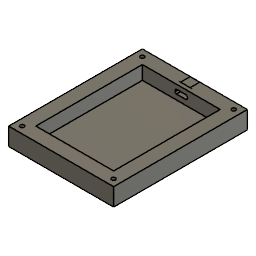
Bottom (Autodesk Fusion 360 design; units mm, degrees)
Autodesk Fusion 360 part; units mm, degrees
sketch "Sketch1" plane through (0, 0, 0) normal (0, 1, 0) x (1, 0, 0)
  line L0 (0, 0) -> (56.985, 0)
  line L1 (56.985, 0) -> (56.985, 78.065)
  line L2 (56.985, 78.065) -> (0, 78.065)
  line L3 (0, 78.065) -> (0, 0)
  line L4 (66.985, -10) -> (66.985, 88.065)
  line L5 (66.985, 88.065) -> (-10, 88.065)
  line L6 (-10, 88.065) -> (-10, -10)
  line L7 (-10, -10) -> (66.985, -10)
  circle A0 centre (-5, 83.065) radius 1.45
  circle A1 centre (-5, -5) radius 1.45
  circle A2 centre (61.985, -5) radius 1.45
  circle A3 centre (61.985, 83.065) radius 1.45
  dimension "d4" = 56.985
  dimension "d5" = 78.065
  dimension "d6" = 10
  dimension "d9" = 2.9
  dimension "d12" = 2.9
  dimension "d15" = 2.9
  dimension "d18" = 2.9
  constraint horizontal L0
  constraint vertical L1
  constraint horizontal L2
  constraint vertical L3
  constraint coincident L0.start L3.end
  measures "d4" distance of L0.start L0.end
  measures "d5" distance of L0.start L2.end
  measures "d9" diameter of A0
  measures "d12" diameter of A1
  measures "d15" diameter of A2
  measures "d18" diameter of A3
extrude "Extrude1" add sketch "Sketch1" along normal blind 3 contours L0 L1 L2 L3 | L4 L5 L6 L7 picked at (18.995, 52.043333) picked at (60.825164, 26.021667) makes body 1
extrude "Extrude2" cut sketch "Sketch1" along normal blind 13 bodies 1
extrude "Extrude3" add sketch "Sketch1" along normal blind 13 bodies 1
move_body "Align1" bodies 1 to x (1, 0, 0) y (0, 1, 0) z (0, 0, 1) at (0, 0, 0)
move_body "Align2" bodies 1 to x (1, 0, 0) y (0, 1, 0) z (0, 0, 1) at (0, 0, 0)
move_body "Align3" bodies 1 to x (1, 0, 0) y (0, 1, 0) z (0, 0, 1) at (-28.4925, -5.248423, 39.0325)
sketch "plate-2026-03-13T21_26_14.409Z" plane through (0, 7.751577, 0) normal (0, 1, 0) x (1, 0, 0)
  line L0 (-25.209257, 35.572548) -> (-12.209257, 35.572548)
  line L1 (-25.209257, 21.572548) -> (-12.209257, 21.572548)
  line L2 (-25.709257, 35.072548) -> (-25.709257, 22.072548)
  line L3 (-11.709257, 35.072548) -> (-11.709257, 22.072548)
  arc A0 (-25.209257, 35.572548) -> (-25.709257, 35.072548) centre (-25.209257, 35.072548) ccw
  arc A1 (-11.709257, 35.072548) -> (-12.209257, 35.572548) centre (-12.209257, 35.072548) ccw
  arc A2 (-25.709257, 22.072548) -> (-25.209257, 21.572548) centre (-25.209257, 22.072548) ccw
  arc A3 (-12.209257, 21.572548) -> (-11.709257, 22.072548) centre (-12.209257, 22.072548) ccw
  line L4 (-6.159257, 35.572548) -> (6.840743, 35.572548)
  line L5 (-6.159257, 21.572548) -> (6.840743, 21.572548)
  line L6 (-6.659257, 35.072548) -> (-6.659257, 22.072548)
  line L7 (7.340743, 35.072548) -> (7.340743, 22.072548)
  arc A4 (-6.159257, 35.572548) -> (-6.659257, 35.072548) centre (-6.159257, 35.072548) ccw
  arc A5 (7.340743, 35.072548) -> (6.840743, 35.572548) centre (6.840743, 35.072548) ccw
  arc A6 (-6.659257, 22.072548) -> (-6.159257, 21.572548) centre (-6.159257, 22.072548) ccw
  arc A7 (6.840743, 21.572548) -> (7.340743, 22.072548) centre (6.840743, 22.072548) ccw
  line L8 (12.890743, 35.572548) -> (25.890743, 35.572548)
  line L9 (12.890743, 21.572548) -> (25.890743, 21.572548)
  line L10 (12.390743, 35.072548) -> (12.390743, 22.072548)
  line L11 (26.390743, 35.072548) -> (26.390743, 22.072548)
  arc A8 (12.890743, 35.572548) -> (12.390743, 35.072548) centre (12.890743, 35.072548) ccw
  arc A9 (26.390743, 35.072548) -> (25.890743, 35.572548) centre (25.890743, 35.072548) ccw
  arc A10 (12.390743, 22.072548) -> (12.890743, 21.572548) centre (12.890743, 22.072548) ccw
  arc A11 (25.890743, 21.572548) -> (26.390743, 22.072548) centre (25.890743, 22.072548) ccw
  line L12 (-25.209257, 16.522548) -> (-12.209257, 16.522548)
  line L13 (-25.209257, 2.522548) -> (-12.209257, 2.522548)
  line L14 (-25.709257, 16.022548) -> (-25.709257, 3.022548)
  line L15 (-11.709257, 16.022548) -> (-11.709257, 3.022548)
  arc A12 (-25.209257, 16.522548) -> (-25.709257, 16.022548) centre (-25.209257, 16.022548) ccw
  arc A13 (-11.709257, 16.022548) -> (-12.209257, 16.522548) centre (-12.209257, 16.022548) ccw
  arc A14 (-25.709257, 3.022548) -> (-25.209257, 2.522548) centre (-25.209257, 3.022548) ccw
  arc A15 (-12.209257, 2.522548) -> (-11.709257, 3.022548) centre (-12.209257, 3.022548) ccw
  line L16 (-6.159257, 16.522548) -> (6.840743, 16.522548)
  line L17 (-6.159257, 2.522548) -> (6.840743, 2.522548)
  line L18 (-6.659257, 16.022548) -> (-6.659257, 3.022548)
  line L19 (7.340743, 16.022548) -> (7.340743, 3.022548)
  arc A16 (-6.159257, 16.522548) -> (-6.659257, 16.022548) centre (-6.159257, 16.022548) ccw
  arc A17 (7.340743, 16.022548) -> (6.840743, 16.522548) centre (6.840743, 16.022548) ccw
  arc A18 (-6.659257, 3.022548) -> (-6.159257, 2.522548) centre (-6.159257, 3.022548) ccw
  arc A19 (6.840743, 2.522548) -> (7.340743, 3.022548) centre (6.840743, 3.022548) ccw
  line L20 (12.890743, 16.522548) -> (25.890743, 16.522548)
  line L21 (12.890743, 2.522548) -> (25.890743, 2.522548)
  line L22 (12.390743, 16.022548) -> (12.390743, 3.022548)
  line L23 (26.390743, 16.022548) -> (26.390743, 3.022548)
  arc A20 (12.890743, 16.522548) -> (12.390743, 16.022548) centre (12.890743, 16.022548) ccw
  arc A21 (26.390743, 16.022548) -> (25.890743, 16.522548) centre (25.890743, 16.022548) ccw
  arc A22 (12.390743, 3.022548) -> (12.890743, 2.522548) centre (12.890743, 3.022548) ccw
  arc A23 (25.890743, 2.522548) -> (26.390743, 3.022548) centre (25.890743, 3.022548) ccw
  line L24 (-25.209257, -2.527452) -> (-12.209257, -2.527452)
  line L25 (-25.209257, -16.527452) -> (-12.209257, -16.527452)
  line L26 (-25.709257, -3.027452) -> (-25.709257, -16.027452)
  line L27 (-11.709257, -3.027452) -> (-11.709257, -16.027452)
  arc A24 (-25.209257, -2.527452) -> (-25.709257, -3.027452) centre (-25.209257, -3.027452) ccw
  arc A25 (-11.709257, -3.027452) -> (-12.209257, -2.527452) centre (-12.209257, -3.027452) ccw
  arc A26 (-25.709257, -16.027452) -> (-25.209257, -16.527452) centre (-25.209257, -16.027452) ccw
  arc A27 (-12.209257, -16.527452) -> (-11.709257, -16.027452) centre (-12.209257, -16.027452) ccw
  line L28 (-6.159257, -2.527452) -> (6.840743, -2.527452)
  line L29 (-6.159257, -16.527452) -> (6.840743, -16.527452)
  line L30 (-6.659257, -3.027452) -> (-6.659257, -16.027452)
  line L31 (7.340743, -3.027452) -> (7.340743, -16.027452)
  arc A28 (-6.159257, -2.527452) -> (-6.659257, -3.027452) centre (-6.159257, -3.027452) ccw
  arc A29 (7.340743, -3.027452) -> (6.840743, -2.527452) centre (6.840743, -3.027452) ccw
  arc A30 (-6.659257, -16.027452) -> (-6.159257, -16.527452) centre (-6.159257, -16.027452) ccw
  arc A31 (6.840743, -16.527452) -> (7.340743, -16.027452) centre (6.840743, -16.027452) ccw
  line L32 (12.890743, -2.527452) -> (25.890743, -2.527452)
  line L33 (12.890743, -16.527452) -> (25.890743, -16.527452)
  line L34 (12.390743, -3.027452) -> (12.390743, -16.027452)
  line L35 (26.390743, -3.027452) -> (26.390743, -16.027452)
  arc A32 (12.890743, -2.527452) -> (12.390743, -3.027452) centre (12.890743, -3.027452) ccw
  arc A33 (26.390743, -3.027452) -> (25.890743, -2.527452) centre (25.890743, -3.027452) ccw
  arc A34 (12.390743, -16.027452) -> (12.890743, -16.527452) centre (12.890743, -16.027452) ccw
  arc A35 (25.890743, -16.527452) -> (26.390743, -16.027452) centre (25.890743, -16.027452) ccw
  line L36 (12.890743, -2.527452) -> (25.890743, -2.527452)
  line L37 (12.890743, -16.527452) -> (25.890743, -16.527452)
  line L38 (12.390743, -3.027452) -> (12.390743, -16.027452)
  line L39 (26.390743, -3.027452) -> (26.390743, -16.027452)
  arc A36 (12.890743, -2.527452) -> (12.390743, -3.027452) centre (12.890743, -3.027452) ccw
  arc A37 (26.390743, -3.027452) -> (25.890743, -2.527452) centre (25.890743, -3.027452) ccw
  arc A38 (12.390743, -16.027452) -> (12.890743, -16.527452) centre (12.890743, -16.027452) ccw
  arc A39 (25.890743, -16.527452) -> (26.390743, -16.027452) centre (25.890743, -16.027452) ccw
  line L40 (-25.209257, -21.577452) -> (-12.209257, -21.577452)
  line L41 (-25.209257, -35.577452) -> (-12.209257, -35.577452)
  line L42 (-25.709257, -22.077452) -> (-25.709257, -35.077452)
  line L43 (-11.709257, -22.077452) -> (-11.709257, -35.077452)
  arc A40 (-25.209257, -21.577452) -> (-25.709257, -22.077452) centre (-25.209257, -22.077452) ccw
  arc A41 (-11.709257, -22.077452) -> (-12.209257, -21.577452) centre (-12.209257, -22.077452) ccw
  arc A42 (-25.709257, -35.077452) -> (-25.209257, -35.577452) centre (-25.209257, -35.077452) ccw
  arc A43 (-12.209257, -35.577452) -> (-11.709257, -35.077452) centre (-12.209257, -35.077452) ccw
  line L44 (-6.159257, -21.577452) -> (6.840743, -21.577452)
  line L45 (-6.159257, -35.577452) -> (6.840743, -35.577452)
  line L46 (-6.659257, -22.077452) -> (-6.659257, -35.077452)
  line L47 (7.340743, -22.077452) -> (7.340743, -35.077452)
  arc A44 (-6.159257, -21.577452) -> (-6.659257, -22.077452) centre (-6.159257, -22.077452) ccw
  arc A45 (7.340743, -22.077452) -> (6.840743, -21.577452) centre (6.840743, -22.077452) ccw
  arc A46 (-6.659257, -35.077452) -> (-6.159257, -35.577452) centre (-6.159257, -35.077452) ccw
  arc A47 (6.840743, -35.577452) -> (7.340743, -35.077452) centre (6.840743, -35.077452) ccw
  line L48 (12.890743, -21.577452) -> (25.890743, -21.577452)
  line L49 (12.890743, -35.577452) -> (25.890743, -35.577452)
  line L50 (12.390743, -22.077452) -> (12.390743, -35.077452)
  line L51 (26.390743, -22.077452) -> (26.390743, -35.077452)
  arc A48 (12.890743, -21.577452) -> (12.390743, -22.077452) centre (12.890743, -22.077452) ccw
  arc A49 (26.390743, -22.077452) -> (25.890743, -21.577452) centre (25.890743, -22.077452) ccw
  arc A50 (12.390743, -35.077452) -> (12.890743, -35.577452) centre (12.890743, -35.077452) ccw
  arc A51 (25.890743, -35.577452) -> (26.390743, -35.077452) centre (25.890743, -35.077452) ccw
  line L52 (-28.234257, -39.156471) -> (28.915743, -39.156471)
  line L53 (-28.234257, 39.046164) -> (28.915743, 39.046164)
  line L54 (-28.234257, -39.156471) -> (-28.234257, 39.046164)
  line L55 (28.915743, -39.156471) -> (28.915743, 39.046164)
move_body "Move1" bodies 1 to x (1, 0, 0) y (0, 1, 0) z (0, 0, 1) at (0.258, 0, 0)
extrude "Extrude4" add sketch "plate-2026-03-13T21_26_14.409Z" 1 faces at (32.590664, 7.751577, 13.010833) along normal blind 3 separate body on bodies 1 makes body 2
sketch "Sketch3" plane through (0, 0, -49.0325) normal (0, 0, -1) x (-1, 0, 0)
  line L0 (-38.7505, -5.248423) -> (38.2345, -5.248423)
  line L1 (38.2345, -5.248423) -> (38.2345, 7.751577)
  line L2 (38.2345, 7.751577) -> (-38.7505, 7.751577)
  line L3 (-38.7505, 7.751577) -> (-38.7505, -5.248423)
  line L4 (-3.758, 1.551577) -> (3.242, 1.551577)
  line L5 (4.242, 2.551577) -> (4.242, 3.551577)
  line L6 (3.242, 4.551577) -> (-3.758, 4.551577)
  line L7 (-4.758, 3.551577) -> (-4.758, 2.551577)
  arc A0 (4.242, 3.551577) -> (3.242, 4.551577) centre (3.242, 3.551577) ccw
  arc A1 (3.242, 1.551577) -> (4.242, 2.551577) centre (3.242, 2.551577) ccw
  arc A2 (-3.758, 4.551577) -> (-4.758, 3.551577) centre (-3.758, 3.551577) ccw
  arc A3 (-4.758, 2.551577) -> (-3.758, 1.551577) centre (-3.758, 2.551577) ccw
  dimension "d34" = 1
  dimension "d35" = 1
  dimension "d36" = 1
  dimension "d37" = 1
  constraint horizontal L4
  constraint vertical L5
  constraint horizontal L6
  constraint vertical L7
  constraint tangent L6 A0
  constraint tangent L5 A0
  constraint tangent L4 A1
  constraint tangent L5 A1
  constraint tangent L7 A2
  constraint tangent L6 A2
  constraint tangent L7 A3
  constraint tangent L4 A3
  measures "d34" radius of A0
  measures "d35" radius of A1
  measures "d36" radius of A2
  measures "d37" radius of A3
extrude "Extrude5" cut sketch "Sketch3" against normal blind 17 contours L4 L5 L6 L7 A0 A1 A2 A3 picked at (0.908667, 2.551577) bodies 1
sketch "Sketch4" plane through (0, 0, -49.0325) normal (0, 0, -1) x (-1, 0, 0)
  line L0 (3.242, 1.551577) -> (-3.758, 1.551577)
  arc A0 (-4.758, 2.551577) -> (-3.758, 1.551577) centre (-3.758, 2.551577) ccw
  line L1 (-4.758, 2.551577) -> (-4.758, 3.551577)
  arc A1 (-3.758, 4.551577) -> (-4.758, 3.551577) centre (-3.758, 3.551577) ccw
  line L2 (-3.758, 4.551577) -> (3.242, 4.551577)
  arc A2 (4.242, 3.551577) -> (3.242, 4.551577) centre (3.242, 3.551577) ccw
  line L3 (4.242, 3.551577) -> (4.242, 2.551577)
  arc A3 (3.242, 1.551577) -> (4.242, 2.551577) centre (3.242, 2.551577) ccw
  line L4 (-38.7505, -5.248423) -> (38.2345, -5.248423)
  line L5 (38.2345, -5.248423) -> (38.2345, 7.751577)
  line L6 (38.2345, 7.751577) -> (-38.7505, 7.751577)
  line L7 (-38.7505, 7.751577) -> (-38.7505, -5.248423)
  arc A4 (7.242, 3.551577) -> (3.242, 7.551577) centre (3.242, 3.551577) ccw
  line L8 (-3.758, 7.551577) -> (3.242, 7.551577)
  arc A5 (-3.758, 7.551577) -> (-7.758, 3.551577) centre (-3.758, 3.551577) ccw
  line L9 (-7.758, 2.551577) -> (-7.758, 3.551577)
  arc A6 (-7.758, 2.551577) -> (-3.758, -1.448423) centre (-3.758, 2.551577) ccw
  line L10 (3.242, -1.448423) -> (-3.758, -1.448423)
  arc A7 (3.242, -1.448423) -> (7.242, 2.551577) centre (3.242, 2.551577) ccw
  line L11 (7.242, 3.551577) -> (7.242, 2.551577)
  dimension "d40" = -3
extrude "Extrude6" cut sketch "Sketch4" against normal blind 7 contours A4 L8 A5 L9 A6 L10 A7 L11 picked at (-1.424667, -0.448423) bodies 1
sketch "Sketch5" plane through (38.7505, 0, 0) normal (1, 0, 0) x (0, 0, -1)
  line L0 (-49.0325, 7.751577) -> (49.0325, 7.751577)
  line L1 (49.0325, 7.751577) -> (49.0325, 10.751577)
  line L2 (49.0325, 10.751577) -> (-49.0325, 10.751577)
  line L3 (-49.0325, 10.751577) -> (-49.0325, 7.751577)
  line L4 (-49.0325, 9.251577) -> (49.0325, 9.251577)
extrude "Extrude7" cut sketch "Sketch5" against normal blind 88 contours L1 L2 L3 L4 picked at (-16.344167, 10.251577) bodies 2
sketch "Sketch6" plane through (0, 9.251577, 0) normal (0, 1, 0) x (-1, 0, 0)
  line L0 (38.2345, -49.0325) -> (38.2345, 49.0325)
  line L1 (38.2345, 49.0325) -> (-38.7505, 49.0325)
  line L2 (-38.7505, 49.0325) -> (-38.7505, -49.0325)
  line L3 (-38.7505, -49.0325) -> (38.2345, -49.0325)
  line L4 (-12.390743, 16.027452) -> (-12.390743, 3.027452)
  arc A0 (-12.890743, 2.527452) -> (-12.390743, 3.027452) centre (-12.890743, 3.027452) ccw
  line L5 (-12.890743, 2.527452) -> (-25.890743, 2.527452)
  arc A1 (-26.390743, 3.027452) -> (-25.890743, 2.527452) centre (-25.890743, 3.027452) ccw
  line L6 (-26.390743, 3.027452) -> (-26.390743, 16.027452)
  arc A2 (-25.890743, 16.527452) -> (-26.390743, 16.027452) centre (-25.890743, 16.027452) ccw
  line L7 (-25.890743, 16.527452) -> (-12.890743, 16.527452)
  arc A3 (-12.390743, 16.027452) -> (-12.890743, 16.527452) centre (-12.890743, 16.027452) ccw
  line L8 (25.709257, -3.022548) -> (25.709257, -16.022548)
  arc A4 (25.209257, -16.522548) -> (25.709257, -16.022548) centre (25.209257, -16.022548) ccw
  line L9 (25.209257, -16.522548) -> (12.209257, -16.522548)
  arc A5 (11.709257, -16.022548) -> (12.209257, -16.522548) centre (12.209257, -16.022548) ccw
  line L10 (11.709257, -16.022548) -> (11.709257, -3.022548)
  arc A6 (12.209257, -2.522548) -> (11.709257, -3.022548) centre (12.209257, -3.022548) ccw
  line L11 (12.209257, -2.522548) -> (25.209257, -2.522548)
  arc A7 (25.709257, -3.022548) -> (25.209257, -2.522548) centre (25.209257, -3.022548) ccw
  line L12 (-12.390743, 35.077452) -> (-12.390743, 22.077452)
  arc A8 (-12.890743, 21.577452) -> (-12.390743, 22.077452) centre (-12.890743, 22.077452) ccw
  line L13 (-12.890743, 21.577452) -> (-25.890743, 21.577452)
  arc A9 (-26.390743, 22.077452) -> (-25.890743, 21.577452) centre (-25.890743, 22.077452) ccw
  line L14 (-26.390743, 22.077452) -> (-26.390743, 35.077452)
  arc A10 (-25.890743, 35.577452) -> (-26.390743, 35.077452) centre (-25.890743, 35.077452) ccw
  line L15 (-25.890743, 35.577452) -> (-12.890743, 35.577452)
  arc A11 (-12.390743, 35.077452) -> (-12.890743, 35.577452) centre (-12.890743, 35.077452) ccw
  line L16 (6.659257, 16.027452) -> (6.659257, 3.027452)
  arc A12 (6.159257, 2.527452) -> (6.659257, 3.027452) centre (6.159257, 3.027452) ccw
  line L17 (6.159257, 2.527452) -> (-6.840743, 2.527452)
  arc A13 (-7.340743, 3.027452) -> (-6.840743, 2.527452) centre (-6.840743, 3.027452) ccw
  line L18 (-7.340743, 3.027452) -> (-7.340743, 16.027452)
  arc A14 (-6.840743, 16.527452) -> (-7.340743, 16.027452) centre (-6.840743, 16.027452) ccw
  line L19 (-6.840743, 16.527452) -> (6.159257, 16.527452)
  arc A15 (6.659257, 16.027452) -> (6.159257, 16.527452) centre (6.159257, 16.027452) ccw
  line L20 (25.709257, 16.027452) -> (25.709257, 3.027452)
  arc A16 (25.209257, 2.527452) -> (25.709257, 3.027452) centre (25.209257, 3.027452) ccw
  line L21 (25.209257, 2.527452) -> (12.209257, 2.527452)
  arc A17 (11.709257, 3.027452) -> (12.209257, 2.527452) centre (12.209257, 3.027452) ccw
  line L22 (11.709257, 3.027452) -> (11.709257, 16.027452)
  arc A18 (12.209257, 16.527452) -> (11.709257, 16.027452) centre (12.209257, 16.027452) ccw
  line L23 (12.209257, 16.527452) -> (25.209257, 16.527452)
  arc A19 (25.709257, 16.027452) -> (25.209257, 16.527452) centre (25.209257, 16.027452) ccw
  line L24 (6.659257, 35.077452) -> (6.659257, 22.077452)
  arc A20 (6.159257, 21.577452) -> (6.659257, 22.077452) centre (6.159257, 22.077452) ccw
  line L25 (6.159257, 21.577452) -> (-6.840743, 21.577452)
  arc A21 (-7.340743, 22.077452) -> (-6.840743, 21.577452) centre (-6.840743, 22.077452) ccw
  line L26 (-7.340743, 22.077452) -> (-7.340743, 35.077452)
  arc A22 (-6.840743, 35.577452) -> (-7.340743, 35.077452) centre (-6.840743, 35.077452) ccw
  line L27 (-6.840743, 35.577452) -> (6.159257, 35.577452)
  arc A23 (6.659257, 35.077452) -> (6.159257, 35.577452) centre (6.159257, 35.077452) ccw
  line L28 (-12.390743, -3.022548) -> (-12.390743, -16.022548)
  arc A24 (-12.890743, -16.522548) -> (-12.390743, -16.022548) centre (-12.890743, -16.022548) ccw
  line L29 (-12.890743, -16.522548) -> (-25.890743, -16.522548)
  arc A25 (-26.390743, -16.022548) -> (-25.890743, -16.522548) centre (-25.890743, -16.022548) ccw
  line L30 (-26.390743, -16.022548) -> (-26.390743, -3.022548)
  arc A26 (-25.890743, -2.522548) -> (-26.390743, -3.022548) centre (-25.890743, -3.022548) ccw
  line L31 (-25.890743, -2.522548) -> (-12.890743, -2.522548)
  arc A27 (-12.390743, -3.022548) -> (-12.890743, -2.522548) centre (-12.890743, -3.022548) ccw
  line L32 (-12.390743, -22.072548) -> (-12.390743, -35.072548)
  arc A28 (-12.890743, -35.572548) -> (-12.390743, -35.072548) centre (-12.890743, -35.072548) ccw
  line L33 (-12.890743, -35.572548) -> (-25.890743, -35.572548)
  arc A29 (-26.390743, -35.072548) -> (-25.890743, -35.572548) centre (-25.890743, -35.072548) ccw
  line L34 (-26.390743, -35.072548) -> (-26.390743, -22.072548)
  arc A30 (-25.890743, -21.572548) -> (-26.390743, -22.072548) centre (-25.890743, -22.072548) ccw
  line L35 (-25.890743, -21.572548) -> (-12.890743, -21.572548)
  arc A31 (-12.390743, -22.072548) -> (-12.890743, -21.572548) centre (-12.890743, -22.072548) ccw
  line L36 (6.659257, -3.022548) -> (6.659257, -16.022548)
  arc A32 (6.159257, -16.522548) -> (6.659257, -16.022548) centre (6.159257, -16.022548) ccw
  line L37 (6.159257, -16.522548) -> (-6.840743, -16.522548)
  arc A33 (-7.340743, -16.022548) -> (-6.840743, -16.522548) centre (-6.840743, -16.022548) ccw
  line L38 (-7.340743, -16.022548) -> (-7.340743, -3.022548)
  arc A34 (-6.840743, -2.522548) -> (-7.340743, -3.022548) centre (-6.840743, -3.022548) ccw
  line L39 (-6.840743, -2.522548) -> (6.159257, -2.522548)
  arc A35 (6.659257, -3.022548) -> (6.159257, -2.522548) centre (6.159257, -3.022548) ccw
  line L40 (25.709257, -22.072548) -> (25.709257, -35.072548)
  arc A36 (25.209257, -35.572548) -> (25.709257, -35.072548) centre (25.209257, -35.072548) ccw
  line L41 (25.209257, -35.572548) -> (12.209257, -35.572548)
  arc A37 (11.709257, -35.072548) -> (12.209257, -35.572548) centre (12.209257, -35.072548) ccw
  line L42 (11.709257, -35.072548) -> (11.709257, -22.072548)
  arc A38 (12.209257, -21.572548) -> (11.709257, -22.072548) centre (12.209257, -22.072548) ccw
  line L43 (12.209257, -21.572548) -> (25.209257, -21.572548)
  arc A39 (25.709257, -22.072548) -> (25.209257, -21.572548) centre (25.209257, -22.072548) ccw
  line L44 (25.709257, 35.077452) -> (25.709257, 22.077452)
  arc A40 (25.209257, 21.577452) -> (25.709257, 22.077452) centre (25.209257, 22.077452) ccw
  line L45 (25.209257, 21.577452) -> (12.209257, 21.577452)
  arc A41 (11.709257, 22.077452) -> (12.209257, 21.577452) centre (12.209257, 22.077452) ccw
  line L46 (11.709257, 22.077452) -> (11.709257, 35.077452)
  arc A42 (12.209257, 35.577452) -> (11.709257, 35.077452) centre (12.209257, 35.077452) ccw
  line L47 (12.209257, 35.577452) -> (25.209257, 35.577452)
  arc A43 (25.709257, 35.077452) -> (25.209257, 35.577452) centre (25.209257, 35.077452) ccw
  line L48 (6.659257, -22.072548) -> (6.659257, -35.072548)
  arc A44 (6.159257, -35.572548) -> (6.659257, -35.072548) centre (6.159257, -35.072548) ccw
  line L49 (6.159257, -35.572548) -> (-6.840743, -35.572548)
  arc A45 (-7.340743, -35.072548) -> (-6.840743, -35.572548) centre (-6.840743, -35.072548) ccw
  line L50 (-7.340743, -35.072548) -> (-7.340743, -22.072548)
  arc A46 (-6.840743, -21.572548) -> (-7.340743, -22.072548) centre (-6.840743, -22.072548) ccw
  line L51 (-6.840743, -21.572548) -> (6.159257, -21.572548)
  arc A47 (6.659257, -22.072548) -> (6.159257, -21.572548) centre (6.159257, -22.072548) ccw
  line L52 (28.234257, 39.0325) -> (28.2345, 39.0325)
  line L53 (28.2345, 39.0325) -> (28.2345, -39.0325)
  line L54 (28.2345, -39.0325) -> (28.234257, -39.0325)
  line L55 (28.234257, -39.0325) -> (28.234257, 39.0325)
  circle A48 centre (33.2345, 44.0325) radius 1.45
  circle A49 centre (-33.7505, -44.0325) radius 1.45
  circle A50 centre (-33.7505, 44.0325) radius 1.45
  circle A51 centre (33.2345, -44.0325) radius 1.45
  line L56 (25.514997, -36.489774) -> (11.914997, -36.489774)
  line L57 (10.914997, -35.489774) -> (10.914997, -21.689774)
  line L58 (26.514997, -35.489774) -> (26.514997, -21.689774)
  line L59 (25.514997, -20.689774) -> (11.914997, -20.689774)
  arc A52 (25.514997, -36.489774) -> (26.514997, -35.489774) centre (25.514997, -35.489774) ccw
  arc A53 (10.914997, -35.489774) -> (11.914997, -36.489774) centre (11.914997, -35.489774) ccw
  arc A54 (11.914997, -20.689774) -> (10.914997, -21.689774) centre (11.914997, -21.689774) ccw
  arc A55 (26.514997, -21.689774) -> (25.514997, -20.689774) centre (25.514997, -21.689774) ccw
  line L60 (6.514997, -36.489774) -> (-7.085003, -36.489774)
  arc A56 (6.514997, -36.489774) -> (7.514997, -35.489774) centre (6.514997, -35.489774) ccw
  line L61 (7.514997, -35.489774) -> (7.514997, -21.689774)
  line L62 (6.514997, -20.689774) -> (-7.085003, -20.689774)
  arc A57 (7.514997, -21.689774) -> (6.514997, -20.689774) centre (6.514997, -21.689774) ccw
  arc A58 (-7.085003, -20.689774) -> (-8.085003, -21.689774) centre (-7.085003, -21.689774) ccw
  line L63 (-8.085003, -35.489774) -> (-8.085003, -21.689774)
  arc A59 (-8.085003, -35.489774) -> (-7.085003, -36.489774) centre (-7.085003, -35.489774) ccw
  line L64 (26.514997, -16.489774) -> (26.514997, -2.689774)
  arc A60 (-7.085003, -1.689774) -> (-8.085003, -2.689774) centre (-7.085003, -2.689774) ccw
  arc A61 (7.514997, -2.689774) -> (6.514997, -1.689774) centre (6.514997, -2.689774) ccw
  arc A62 (25.514997, -17.489774) -> (26.514997, -16.489774) centre (25.514997, -16.489774) ccw
  arc A63 (11.914997, -1.689774) -> (10.914997, -2.689774) centre (11.914997, -2.689774) ccw
  arc A64 (10.914997, -16.489774) -> (11.914997, -17.489774) centre (11.914997, -16.489774) ccw
  line L65 (6.514997, -1.689774) -> (-7.085003, -1.689774)
  arc A65 (26.514997, -2.689774) -> (25.514997, -1.689774) centre (25.514997, -2.689774) ccw
  line L66 (25.514997, -1.689774) -> (11.914997, -1.689774)
  arc A66 (-8.085003, -16.489774) -> (-7.085003, -17.489774) centre (-7.085003, -16.489774) ccw
  line L67 (10.914997, -16.489774) -> (10.914997, -2.689774)
  arc A67 (6.514997, -17.489774) -> (7.514997, -16.489774) centre (6.514997, -16.489774) ccw
  line L68 (-8.085003, -16.489774) -> (-8.085003, -2.689774)
  line L69 (7.514997, -16.489774) -> (7.514997, -2.689774)
  line L70 (6.514997, -17.489774) -> (-7.085003, -17.489774)
  line L71 (25.514997, -17.489774) -> (11.914997, -17.489774)
  arc A68 (-26.085003, -20.689774) -> (-27.085003, -21.689774) centre (-26.085003, -21.689774) ccw
  arc A69 (-11.485003, -21.689774) -> (-12.485003, -20.689774) centre (-12.485003, -21.689774) ccw
  arc A70 (-27.085003, -35.489774) -> (-26.085003, -36.489774) centre (-26.085003, -35.489774) ccw
  line L72 (-11.485003, -35.489774) -> (-11.485003, -21.689774)
  line L73 (-27.085003, -35.489774) -> (-27.085003, -21.689774)
  line L74 (-12.485003, -36.489774) -> (-26.085003, -36.489774)
  line L75 (-12.485003, -20.689774) -> (-26.085003, -20.689774)
  arc A71 (-12.485003, -36.489774) -> (-11.485003, -35.489774) centre (-12.485003, -35.489774) ccw
  arc A72 (-26.085003, -1.689774) -> (-27.085003, -2.689774) centre (-26.085003, -2.689774) ccw
  arc A73 (-12.485003, -17.489774) -> (-11.485003, -16.489774) centre (-12.485003, -16.489774) ccw
  line L76 (-12.485003, -1.689774) -> (-26.085003, -1.689774)
  arc A74 (-27.085003, -16.489774) -> (-26.085003, -17.489774) centre (-26.085003, -16.489774) ccw
  line L77 (-27.085003, -16.489774) -> (-27.085003, -2.689774)
  arc A75 (-11.485003, -2.689774) -> (-12.485003, -1.689774) centre (-12.485003, -2.689774) ccw
  line L78 (-11.485003, -16.489774) -> (-11.485003, -2.689774)
  line L79 (-12.485003, -17.489774) -> (-26.085003, -17.489774)
  arc A76 (-26.085003, 17.310226) -> (-27.085003, 16.310226) centre (-26.085003, 16.310226) ccw
  line L80 (-27.085003, 2.510226) -> (-27.085003, 16.310226)
  line L81 (-12.485003, 1.510226) -> (-26.085003, 1.510226)
  line L82 (6.514997, 17.310226) -> (-7.085003, 17.310226)
  line L83 (-8.085003, 21.510226) -> (-8.085003, 35.310226)
  arc A77 (-12.485003, 1.510226) -> (-11.485003, 2.510226) centre (-12.485003, 2.510226) ccw
  arc A78 (-27.085003, 2.510226) -> (-26.085003, 1.510226) centre (-26.085003, 2.510226) ccw
  arc A79 (-8.085003, 2.510226) -> (-7.085003, 1.510226) centre (-7.085003, 2.510226) ccw
  arc A80 (-8.085003, 21.510226) -> (-7.085003, 20.510226) centre (-7.085003, 21.510226) ccw
  line L84 (-12.485003, 17.310226) -> (-26.085003, 17.310226)
  line L85 (6.514997, 36.310226) -> (-7.085003, 36.310226)
  arc A81 (-11.485003, 16.310226) -> (-12.485003, 17.310226) centre (-12.485003, 16.310226) ccw
  arc A82 (-7.085003, 17.310226) -> (-8.085003, 16.310226) centre (-7.085003, 16.310226) ccw
  arc A83 (6.514997, 1.510226) -> (7.514997, 2.510226) centre (6.514997, 2.510226) ccw
  arc A84 (-7.085003, 36.310226) -> (-8.085003, 35.310226) centre (-7.085003, 35.310226) ccw
  line L86 (-11.485003, 2.510226) -> (-11.485003, 16.310226)
  line L87 (26.514997, 21.510226) -> (26.514997, 35.310226)
  line L88 (7.514997, 2.510226) -> (7.514997, 16.310226)
  line L89 (7.514997, 21.510226) -> (7.514997, 35.310226)
  line L90 (25.514997, 17.310226) -> (11.914997, 17.310226)
  arc A85 (25.514997, 1.510226) -> (26.514997, 2.510226) centre (25.514997, 2.510226) ccw
  line L91 (25.514997, 20.510226) -> (11.914997, 20.510226)
  arc A86 (11.914997, 36.310226) -> (10.914997, 35.310226) centre (11.914997, 35.310226) ccw
  line L92 (10.914997, 2.510226) -> (10.914997, 16.310226)
  line L93 (25.514997, 36.310226) -> (11.914997, 36.310226)
  arc A87 (11.914997, 17.310226) -> (10.914997, 16.310226) centre (11.914997, 16.310226) ccw
  arc A88 (10.914997, 2.510226) -> (11.914997, 1.510226) centre (11.914997, 2.510226) ccw
  arc A89 (25.514997, 20.510226) -> (26.514997, 21.510226) centre (25.514997, 21.510226) ccw
  arc A90 (10.914997, 21.510226) -> (11.914997, 20.510226) centre (11.914997, 21.510226) ccw
  arc A91 (26.514997, 35.310226) -> (25.514997, 36.310226) centre (25.514997, 35.310226) ccw
  arc A92 (26.514997, 16.310226) -> (25.514997, 17.310226) centre (25.514997, 16.310226) ccw
  line L94 (10.914997, 21.510226) -> (10.914997, 35.310226)
  line L95 (25.514997, 1.510226) -> (11.914997, 1.510226)
  arc A93 (-27.085003, 21.510226) -> (-26.085003, 20.510226) centre (-26.085003, 21.510226) ccw
  arc A94 (-12.485003, 20.510226) -> (-11.485003, 21.510226) centre (-12.485003, 21.510226) ccw
  line L96 (26.514997, 2.510226) -> (26.514997, 16.310226)
  line L97 (-11.485003, 21.510226) -> (-11.485003, 35.310226)
  line L98 (-12.485003, 36.310226) -> (-26.085003, 36.310226)
  arc A95 (-11.485003, 35.310226) -> (-12.485003, 36.310226) centre (-12.485003, 35.310226) ccw
  line L99 (-12.485003, 20.510226) -> (-26.085003, 20.510226)
  arc A96 (-26.085003, 36.310226) -> (-27.085003, 35.310226) centre (-26.085003, 35.310226) ccw
  line L100 (-27.085003, 21.510226) -> (-27.085003, 35.310226)
  line L101 (-8.085003, 2.510226) -> (-8.085003, 16.310226)
  arc A97 (7.514997, 35.310226) -> (6.514997, 36.310226) centre (6.514997, 35.310226) ccw
  line L102 (6.514997, 1.510226) -> (-7.085003, 1.510226)
  arc A98 (6.514997, 20.510226) -> (7.514997, 21.510226) centre (6.514997, 21.510226) ccw
  arc A99 (7.514997, 16.310226) -> (6.514997, 17.310226) centre (6.514997, 16.310226) ccw
  line L103 (6.514997, 20.510226) -> (-7.085003, 20.510226)
  point P0 (26.514997, -36.489774)
  point P1 (10.914997, -36.489774)
  point P2 (10.914997, -20.689774)
  point P3 (10.914997, -1.689774)
  point P4 (26.514997, -17.489774)
  point P5 (10.914997, -17.489774)
  point P6 (10.914997, 17.310226)
  point P7 (26.514997, 1.510226)
  point P8 (10.914997, 1.510226)
  point P9 (10.914997, 36.310226)
  point P10 (26.514997, 20.510226)
  point P11 (10.914997, 20.510226)
  dimension "d45" = 15.6
  dimension "d46" = 15.8
  dimension "d47" = 1
  dimension "d48" = 1
  dimension "d49" = 1
  dimension "d50" = 1
  dimension "d51" = 1
  dimension "d52" = 1
  dimension "d53" = 1
  dimension "d54" = 1
  dimension "d55" = 15.6
  dimension "d56" = 15.8
  dimension "d57" = 1
  dimension "d58" = 1
  dimension "d59" = 1
  dimension "d60" = 1
  dimension "d61" = 1
  dimension "d62" = 1
  dimension "d63" = 1
  dimension "d64" = 1
  dimension "d65" = 1
  dimension "d66" = 1
  dimension "d67" = 1
  dimension "d68" = 1
  dimension "d69" = 1
  dimension "d70" = 1
  dimension "d71" = 1
  dimension "d72" = 1
  dimension "d73" = 15.6
  dimension "d74" = 15.8
  dimension "d75" = 1
  dimension "d76" = 1
  dimension "d77" = 1
  dimension "d78" = 1
  dimension "d79" = 1
  dimension "d80" = 1
  dimension "d81" = 1
  dimension "d82" = 1
  dimension "d83" = 15.6
  dimension "d84" = 15.8
  dimension "d85" = 1
  dimension "d86" = 1
  dimension "d87" = 1
  dimension "d88" = 1
  dimension "d89" = 1
  dimension "d90" = 1
  dimension "d91" = 1
  dimension "d92" = 1
  dimension "d93" = 1
  dimension "d94" = 1
  dimension "d95" = 1
  dimension "d96" = 1
  dimension "d97" = 1
  dimension "d98" = 1
  dimension "d99" = 1
  dimension "d100" = 1
  constraint perpendicular L40 L56
  constraint perpendicular L56 L57
  constraint perpendicular L56 L58
  constraint perpendicular L57 L59
  constraint tangent L56 A52
  constraint tangent L58 A52
  constraint tangent L56 A53
  constraint tangent L57 A53
  constraint tangent L59 A54
  constraint tangent L57 A54
  constraint tangent L58 A55
  constraint tangent L59 A55
  constraint perpendicular L60 L63
  constraint perpendicular L60 L61
  constraint perpendicular L62 L63
  constraint tangent L60 A56
  constraint tangent A56 L61
  constraint tangent L60 A59
  constraint tangent L63 A59
  constraint tangent L62 A58
  constraint tangent A58 L63
  constraint tangent L61 A57
  constraint tangent L62 A57
  constraint perpendicular L67 L71
  constraint perpendicular L64 L71
  constraint perpendicular L66 L67
  constraint tangent A62 L71
  constraint tangent L64 A62
  constraint tangent A64 L71
  constraint tangent A64 L67
  constraint tangent A63 L66
  constraint tangent A63 L67
  constraint tangent L64 A65
  constraint tangent A65 L66
  constraint perpendicular L68 L70
  constraint perpendicular L69 L70
  constraint perpendicular L65 L68
  constraint tangent A67 L70
  constraint tangent A67 L69
  constraint tangent A66 L70
  constraint tangent A66 L68
  constraint tangent A60 L65
  constraint tangent A60 L68
  constraint tangent A61 L69
  constraint tangent A61 L65
  constraint perpendicular L73 L74
  constraint perpendicular L72 L74
  constraint perpendicular L73 L75
  constraint tangent L74 A71
  constraint tangent L72 A71
  constraint tangent A70 L74
  constraint tangent A70 L73
  constraint tangent A68 L75
  constraint tangent A68 L73
  constraint tangent A69 L72
  constraint tangent A69 L75
  constraint perpendicular L77 L79
  constraint perpendicular L78 L79
  constraint perpendicular L76 L77
  constraint tangent A73 L79
  constraint tangent A73 L78
  constraint tangent A74 L79
  constraint tangent A74 L77
  constraint tangent A72 L76
  constraint tangent A72 L77
  constraint tangent A75 L78
  constraint tangent L76 A75
  constraint perpendicular L92 L95
  constraint perpendicular L95 L96
  constraint perpendicular L90 L92
  constraint tangent A85 L95
  constraint tangent A85 L96
  constraint tangent A88 L95
  constraint tangent L92 A88
  constraint tangent L90 A87
  constraint tangent L92 A87
  constraint tangent A92 L96
  constraint tangent L90 A92
  constraint perpendicular L101 L102
  constraint perpendicular L88 L102
  constraint perpendicular L82 L101
  constraint tangent A83 L102
  constraint tangent A83 L88
  constraint tangent A79 L102
  constraint tangent A79 L101
  constraint tangent L82 A82
  constraint tangent A82 L101
  constraint tangent L88 A99
  constraint tangent L82 A99
  constraint perpendicular L91 L94
  constraint perpendicular L87 L91
  constraint perpendicular L93 L94
  constraint tangent L91 A89
  constraint tangent L87 A89
  constraint tangent L91 A90
  constraint tangent A90 L94
  constraint tangent A86 L93
  constraint tangent A86 L94
  constraint tangent L87 A91
  constraint tangent L93 A91
  constraint perpendicular L83 L103
  constraint perpendicular L89 L103
  constraint perpendicular L83 L85
  constraint tangent A98 L103
  constraint tangent L89 A98
  constraint tangent A80 L103
  constraint tangent L83 A80
  constraint tangent L85 A84
  constraint tangent L83 A84
  constraint tangent L89 A97
  constraint tangent L85 A97
  constraint perpendicular L80 L81
  constraint perpendicular L81 L86
  constraint perpendicular L80 L84
  constraint tangent L81 A77
  constraint tangent A77 L86
  constraint tangent L81 A78
  constraint tangent L80 A78
  constraint tangent A76 L84
  constraint tangent A76 L80
  constraint tangent A81 L86
  constraint tangent L84 A81
  constraint perpendicular L99 L100
  constraint perpendicular L97 L99
  constraint perpendicular L98 L100
  constraint tangent A94 L99
  constraint tangent A94 L97
  constraint tangent A93 L99
  constraint tangent A93 L100
  constraint tangent L98 A96
  constraint tangent A96 L100
  constraint tangent L97 A95
  constraint tangent L98 A95
  measures "d47" radius of A52
  measures "d48" radius of A53
  measures "d49" radius of A54
  measures "d50" radius of A55
  measures "d51" radius of A56
  measures "d52" radius of A59
  measures "d53" radius of A58
  measures "d54" radius of A57
  measures "d57" radius of A62
  measures "d58" radius of A64
  measures "d59" radius of A63
  measures "d60" radius of A65
  measures "d61" radius of A67
  measures "d62" radius of A66
  measures "d63" radius of A60
  measures "d64" radius of A61
  measures "d65" radius of A71
  measures "d66" radius of A70
  measures "d67" radius of A68
  measures "d68" radius of A69
  measures "d69" radius of A73
  measures "d70" radius of A74
  measures "d71" radius of A72
  measures "d72" radius of A75
  measures "d75" radius of A85
  measures "d76" radius of A88
  measures "d77" radius of A87
  measures "d78" radius of A92
  measures "d79" radius of A83
  measures "d80" radius of A79
  measures "d81" radius of A82
  measures "d82" radius of A99
  measures "d85" radius of A89
  measures "d86" radius of A90
  measures "d87" radius of A86
  measures "d88" radius of A91
  measures "d89" radius of A98
  measures "d90" radius of A80
  measures "d91" radius of A84
  measures "d92" radius of A97
  measures "d93" radius of A77
  measures "d94" radius of A78
  measures "d95" radius of A76
  measures "d96" radius of A81
  measures "d97" radius of A94
  measures "d98" radius of A93
  measures "d99" radius of A96
  measures "d100" radius of A95
extrude "Extrude8" cut sketch "Sketch6" against normal blind 6 contours L56 L57 L58 L59 A52 A53 A54 A55 | L60 A56 L61 L62 A57 A58 L63 A59 | L64 A62 A63 A64 A65 L66 L67 L71 | A60 A61 L65 A66 A67 L68 L69 L70 | A68 A69 A70 L72 L73 L74 L75 A71 | A72 A73 L76 A74 L77 A75 L78 L79 | A76 L80 L81 A77 A78 L84 A81 L86 | L82 A79 A82 A83 L88 L101 L102 A99 | L83 A80 L85 A84 L89 A97 A98 L103 | L87 L91 A86 L93 A89 A90 A91 L94 | L90 A85 L92 A87 A88 A92 L95 L96 | A93 A94 L97 L98 A95 L99 A96 L100 picked at (20.87975, -36.184032) picked at (1.863083, -36.184032) picked at (20.87975, -17.167365) picked at (1.863083, -17.167365) picked at (-17.153583, -36.184032) picked at (-17.153583, -17.167365) picked at (-17.153583, 1.849301) picked at (1.863083, 1.849301) picked at (1.863083, 20.865968) picked at (20.87975, 20.865968) picked at (20.87975, 1.849301) picked at (-17.153583, 20.865968) bodies 2
hidden bodies 2
